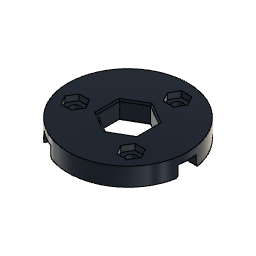
Picavet_supportgodetbas v5 (Autodesk Fusion 360 design; units mm, degrees)
Autodesk Fusion 360 part; units mm, degrees
sketch "Esquisse1" plane through (0, 0, 0) normal (0, 0, 1) x (1, 0, 0)
  circle A0 centre (0, 0) radius 20
  line L0 (19.7661, -3.05) -> (8.2661, -3.05)
  line L1 (8.2661, -3.05) -> (8.2661, 3.1)
  line L2 (14.3661, 3.05) -> (19.7661, 3.05)
  line L3 (8.2661, -3.05) -> (14.4604, -3.05)
  line L4 (14.3661, 10.35) -> (8.2661, 10.35)
  line L5 (8.2661, 10.35) -> (8.2661, -3.05)
  line L6 (0, 0) -> (29, 0) construction
  line L7 (14.3661, 3.05) -> (14.3661, 10.35)
  line L8 (-9.8244, 10.9164) -> (-16.1464, 7.2664)
  line L9 (-16.1464, 7.2664) -> (-13.0964, 1.9836)
  line L10 (-13.0964, 1.9836) -> (-1.4917, 8.6836)
  line L11 (-1.4917, 8.6836) -> (-4.5888, 14.0481)
  line L12 (-7.2417, 18.6429) -> (-1.4917, 8.6836)
  line L13 (-9.8244, 10.9164) -> (-12.5244, 15.5929)
  line L14 (-4.5417, -13.9664) -> (1.7803, -17.6164)
  line L15 (1.7803, -17.6164) -> (4.8303, -12.3336)
  line L16 (4.8303, -12.3336) -> (-6.7744, -5.6336)
  line L17 (-6.7744, -5.6336) -> (-9.8716, -10.9981)
  line L18 (-12.5244, -15.5929) -> (-6.7744, -5.6336)
  line L19 (-4.5417, -13.9664) -> (-7.2417, -18.6429)
  circle A1 centre (2.9108, 13.6941) radius 1.75
  line L20 (0, 0) -> (2.9108, 13.6941) construction
  circle A2 centre (-13.3148, -4.3262) radius 1.75
  circle A3 centre (10.404, -9.3678) radius 1.75
  line L21 (0, 7.5633) -> (-6.55, 3.7816)
  line L22 (-6.55, 3.7816) -> (-6.55, -3.7816)
  line L23 (-6.55, -3.7816) -> (0, -7.5633)
  line L24 (0, -7.5633) -> (6.55, -3.7816)
  line L25 (6.55, -3.7816) -> (6.55, 3.7816)
  line L26 (6.55, 3.7816) -> (0, 7.5633)
  dimension "d1" = 40
  dimension "d2" = 6.1
  dimension "d3" = 11.5
  dimension "d6" = 6.1
  dimension "d7" = 3.05
  dimension "d8" = 13.4
  dimension "d10" = 360
  dimension "d16" = 3.5
  dimension "d17" = 78
  dimension "d19" = 360
  dimension "d21" = 14
  dimension "d25" = 6.55
  constraint coincident A0.centre L6.start
  constraint horizontal L0
  constraint vertical L1
  constraint horizontal L2
  constraint coincident A0 L0.start
  constraint coincident A0 L2.end
  constraint horizontal L3
  constraint horizontal L4
  constraint vertical L5
  constraint horizontal L6
  constraint perpendicular L2 L7
  constraint coincident A1.centre L20.end
  constraint parallel L1 L25
  measures "d1" diameter of A0
  measures "d2" distance of L0.start L2.end
  measures "d3" distance of L0.start L0.end
  measures "d6" distance of L4.start L4.end
  measures "d7" distance of L2 L6
  measures "d8" distance of L0.end L4.end
  measures "d16" diameter of A1
  measures "d17" angle of L6 L20
  measures "d21" distance of A0.centre A1.centre
  measures "d25" distance of A0.centre L26
extrude "Extrusion1" add sketch "Esquisse1" along normal blind 6.1 contours A0 L0 L1 L2 L3 L4 L5 L7 | A0 L0 L1 L2 L3 L4 L5 L7 L8 L9 L10 L11 L12 L13 L14 L15 L16 L17 L18 L19 | A0 L8 L9 L10 L11 L12 L13 | A0 L14 L15 L16 L17 L18 L19 | A1 | A2 | A3 | L21 L22 L23 L24 L25 L26
extrude "Extrusion2" cut sketch "Esquisse1" along normal blind 3.7 contours A0 L0 L1 L2 L3 L4 L5 L7 | A0 L8 L9 L10 L11 L12 L13 | A0 L14 L15 L16 L17 L18 L19
extrude "Extrusion3" cut sketch "Esquisse1" along normal blind 6.1 contours A1 | A2 | A3
chamfer "Chanfrein1" distance 0.5 angle 45 15 edges at (-4.3667, 13.6633, 0) (-11.1744, 13.2546, 0) (-12.9854, 9.0914, 0) (-14.6214, 4.625, 0) (-7.294, 5.3336, 0) (-9.6494, -10.6133, 0) (-0.972, -8.9836, 0) (-5.8917, -16.3046, 0) (-1.3807, -15.7914, 0) (3.3053, -14.975, 0) (8.2661, 3.65, 0) (14.0161, -3.05, 0) (17.0661, 3.05, 0) (14.3661, 6.7, 0) (11.3161, 10.35, 0)
extrude "Extrusion4" cut sketch "Esquisse1" along normal blind 6.1 contours L21 L22 L23 L24 L25 L26
chamfer "Chanfrein2" distance 0.5 angle 45 6 edges at (-3.275, -5.6725, 6.1) (-6.55, 0, 6.1) (-3.275, 5.6725, 6.1) (3.275, 5.6725, 6.1) (6.55, 0, 6.1) (3.275, -5.6725, 6.1)
chamfer "Chanfrein3" distance 0.5 angle 45 6 edges at (-6.55, 0, 0) (-3.275, -5.6725, 0) (3.275, -5.6725, 0) (6.55, 0, 0) (3.275, 5.6725, 0) (-3.275, 5.6725, 0)
sketch "Esquisse3" plane through (0, 0, 6.1) normal (0, 0, 1) x (-1, 0, 0)
  circle A0 centre (0, 0) radius 20
  circle A1 centre (-2.9108, -13.6941) radius 1.75
  circle A2 centre (13.3148, 4.3262) radius 1.75
  circle A3 centre (-10.404, 9.3678) radius 1.75
  line L0 (-7.05, -4.0703) -> (-7.05, 4.0703)
  line L1 (-7.05, 4.0703) -> (0, 8.1406)
  line L2 (0, 8.1406) -> (7.05, 4.0703)
  line L3 (7.05, 4.0703) -> (7.05, -4.0703)
  line L4 (7.05, -4.0703) -> (0, -8.1406)
  line L5 (0, -8.1406) -> (-7.05, -4.0703)
  line L6 (-4.6428, -10.6941) -> (-6.3749, -13.6941)
  line L7 (-6.3749, -13.6941) -> (-4.6428, -16.6941)
  line L8 (-4.6428, -16.6941) -> (-1.1787, -16.6941)
  line L9 (-1.1787, -16.6941) -> (0.5533, -13.6941)
  line L10 (0.5533, -13.6941) -> (-1.1787, -10.6941)
  line L11 (-1.1787, -10.6941) -> (-4.6428, -10.6941)
  line L12 (9.8507, 4.3262) -> (11.5827, 1.3262)
  line L13 (11.5827, 7.3262) -> (9.8507, 4.3262)
  line L14 (15.0468, 7.3262) -> (11.5827, 7.3262)
  line L15 (16.7789, 4.3262) -> (15.0468, 7.3262)
  line L16 (15.0468, 1.3262) -> (16.7789, 4.3262)
  line L17 (11.5827, 1.3262) -> (15.0468, 1.3262)
  line L18 (-8.672, 6.3678) -> (-6.9399, 9.3678)
  line L19 (-12.1361, 6.3678) -> (-8.672, 6.3678)
  line L20 (-13.8681, 9.3678) -> (-12.1361, 6.3678)
  line L21 (-12.1361, 12.3678) -> (-13.8681, 9.3678)
  line L22 (-8.672, 12.3678) -> (-12.1361, 12.3678)
  line L23 (-6.9399, 9.3678) -> (-8.672, 12.3678)
  point P0 (-2.9108, -13.6941)
  dimension "d30" = 3
  dimension "d32" = 360
  constraint coincident P0 A1.centre
  measures "d30" distance of P0 L11
extrude "Extrusion5" cut sketch "Esquisse3" against normal blind 2 contours L6 L7 L8 L9 L10 L11 | L12 L13 L14 L15 L16 L17 | L18 L19 L20 L21 L22 L23
equation "d6 = d2"
equation "d7 = d2 / 2"
